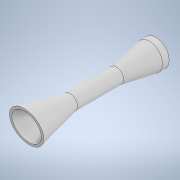
# Autodesk Inventor part: Weapon-Projectile-Stock
Saved by Autodesk Inventor 2020 (Build 240168000, 168)
## iProperties
Created: 2019-11-12
Part Number: Weapon-Projectile-Stock
Material: Generic
Document SubType Name: Modeling
Designer: Victor
Density: 1 g/cm^3
Appearance: Default
Author: Victor
Autodesk Inventor part; units mm, degrees
ref_plane "YZ Plane" through (0, 0, 0) normal (1, 0, 0) x (0, 1, 0)
ref_plane "XZ Plane" through (0, 0, 0) normal (0, 1, 0) x (-1, 0, 0)
ref_plane "XY Plane" through (0, 0, 0) normal (0, 0, 1) x (1, 0, 0)
sketch "Sketch1" plane through (0, 0, 0) normal (0, 0, 1) x (1, 0, 0)
  circle A0 centre (0, 0) radius 10
  dimension "d0" = 20
  constraints: 1 centre point, 1 coincident
  measures "d0" diameter of A0
extrude "Extrusion1" add sketch "Sketch1" along normal blind 5
sketch "Sketch3" plane through (0, 0, 5) normal (0, 0, 1) x (1, 0, 0)
  circle A0 centre (0, 0) radius 10
  constraints: 1 centre point, 1 coincident
extrude "Extrusion3" add sketch "Sketch3" along normal blind 25 draft -10
sketch "Sketch4" plane through (0, 0, 30) normal (0, 0, 1) x (1, 0, 0)
  circle A0 centre (0, 0) radius 5.5918
  constraints: 1 centre point, 1 coincident
extrude "Extrusion4" add sketch "Sketch4" along normal blind 35
sketch "Sketch5" plane through (0, 0, 65) normal (0, 0, 1) x (1, 0, 0)
  circle A0 centre (0, 0) radius 5.5918
  constraints: 1 centre point, 1 coincident
extrude "Extrusion5" add sketch "Sketch5" along normal blind 35 draft 12.5
ref_plane "Work Plane1" through (0, 0, 100) normal (0, 0, 1) x (1, 0, 0)
sketch "Sketch6" plane through (0, 0, 0) normal (1, 0, 0) x (0, 1, 0)
  line L0 (5.5918, 65) -> (13.3511, 100) projected
  line L1 (13.3511, 100) -> (-12.4801, 96.0711)
  line L2 (-5.5918, 65) -> (-13.3511, 100) projected
  line L3 (-13.3511, 100) -> (13.3511, 100) projected
  line L4 (-13.3511, 100) -> (-12.4801, 96.0711)
  line L5 (-13.3511, 100) -> (13.3511, 100)
  point P0 (0, 0)
  constraints: 6 end point, 2 point on line, 1 horizontal
extrude "Extrusion6" cut sketch "Sketch6" along normal mid plane 35
sketch "Sketch7" plane through (0, 0, 100) normal (0, 0, 1) x (1, 0, 0)
  circle A0 centre (0, 0) radius 11.5
  dimension "d16" = 23
  constraints: 1 centre point, 1 coincident
  measures "d16" diameter of A0
extrude "Extrusion7" cut sketch "Sketch7" against normal blind 35 draft -12.5
body "Solid1"
